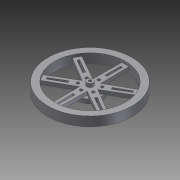
# Autodesk Inventor part: Wheel90mm
Saved by Autodesk Inventor 2011 SP2 (Build 150309200, 309)
## iProperties
Created: 2015-10-13
Part Number: Wheel90mm
Document SubType Name: Modeling
Designer: Ernest
Density: 1 g/cm^3
Author: Ernest
Autodesk Inventor part; units mm, degrees
ref_plane "YZ Plane" through (0, 0, 0) normal (1, 0, 0) x (0, 1, 0)
ref_plane "XZ Plane" through (0, 0, 0) normal (0, 1, 0) x (-1, 0, 0)
ref_plane "XY Plane" through (0, 0, 0) normal (0, 0, 1) x (1, 0, 0)
sketch "Sketch1" plane through (0, 0, 0) normal (0, 0, 1) x (1, 0, 0)
  circle A0 centre (0, 0) radius 45
  circle A1 centre (0, 0) radius 38
  line L0 (0, 0) -> (0, -38) construction
  line L1 (-1.25, -17) -> (1.25, -17)
  line L2 (1.25, -17) -> (1.05, -34)
  line L3 (1.05, -34) -> (-1.05, -34)
  line L4 (-1.25, -17) -> (-1.05, -34)
  circle A2 centre (0, 0) radius 1.5
  circle A3 centre (0, -9.53) radius 1.6035
  circle A4 centre (8.2532, -4.765) radius 1.6035
  circle A5 centre (8.2532, 4.765) radius 1.6035
  circle A6 centre (0, 9.53) radius 1.6035
  circle A7 centre (-8.2532, 4.765) radius 1.6035
  circle A8 centre (-8.2532, -4.765) radius 1.6035
  line L5 (0, -9.53) -> (8.2532, -4.765) construction
  line L6 (4.1266, -7.1475) -> (3.7658, -37.8129)
  line L7 (0, -9.53) -> (-8.2532, -4.765) construction
  line L8 (-4.1266, -7.1475) -> (-3.7658, -37.8129)
  line L9 (14.0974, -9.5825) -> (15.3474, -7.4175)
  line L10 (15.3474, -7.4175) -> (29.9699, -16.0907)
  line L11 (29.9699, -16.0907) -> (28.9199, -17.9093)
  line L12 (14.0974, -9.5825) -> (28.9199, -17.9093)
  line L13 (8.2532, 0) -> (34.6299, -15.6452)
  line L14 (4.1266, -7.1475) -> (30.864, -22.1678)
  line L15 (15.3474, 7.4175) -> (14.0974, 9.5825)
  line L16 (14.0974, 9.5825) -> (28.9199, 17.9093)
  line L17 (28.9199, 17.9093) -> (29.9699, 16.0907)
  line L18 (15.3474, 7.4175) -> (29.9699, 16.0907)
  line L19 (4.1266, 7.1475) -> (30.864, 22.1678)
  line L20 (8.2532, 0) -> (34.6299, 15.6452)
  line L21 (1.25, 17) -> (-1.25, 17)
  line L22 (-1.25, 17) -> (-1.05, 34)
  line L23 (-1.05, 34) -> (1.05, 34)
  line L24 (1.25, 17) -> (1.05, 34)
  line L25 (-4.1266, 7.1475) -> (-3.7658, 37.8129)
  line L26 (4.1266, 7.1475) -> (3.7658, 37.8129)
  line L27 (-14.0974, 9.5825) -> (-15.3474, 7.4175)
  line L28 (-15.3474, 7.4175) -> (-29.9699, 16.0907)
  line L29 (-29.9699, 16.0907) -> (-28.9199, 17.9093)
  line L30 (-14.0974, 9.5825) -> (-28.9199, 17.9093)
  line L31 (-8.2532, 0) -> (-34.6299, 15.6452)
  line L32 (-4.1266, 7.1475) -> (-30.864, 22.1678)
  line L33 (-15.3474, -7.4175) -> (-14.0974, -9.5825)
  line L34 (-14.0974, -9.5825) -> (-28.9199, -17.9093)
  line L35 (-28.9199, -17.9093) -> (-29.9699, -16.0907)
  line L36 (-15.3474, -7.4175) -> (-29.9699, -16.0907)
  line L37 (-4.1266, -7.1475) -> (-30.864, -22.1678)
  line L38 (-8.2532, 0) -> (-34.6299, -15.6452)
  line L39 (3.7658, -37.8129) -> (4.1266, -7.1475)
  line L40 (30.864, -22.1678) -> (4.1266, -7.1475)
  arc A9 (-30.864, -22.1678) -> (-3.7658, -37.8129) centre (0, 0) ccw
  arc A10 (3.7658, -37.8129) -> (30.864, -22.1678) centre (0, 0) ccw
  line L41 (-30.864, -22.1678) -> (-4.1266, -7.1475)
  line L42 (-4.1266, -7.1475) -> (-3.7658, -37.8129)
  line L43 (-34.6299, -15.6452) -> (-8.2532, 0)
  line L44 (-34.6299, 15.6452) -> (-8.2532, 0)
  line L45 (-4.1266, 7.1475) -> (-30.864, 22.1678)
  line L46 (-4.1266, 7.1475) -> (-3.7658, 37.8129)
  line L47 (4.1266, 7.1475) -> (3.7658, 37.8129)
  line L48 (4.1266, 7.1475) -> (30.864, 22.1678)
  line L49 (34.6299, 15.6452) -> (8.2532, 0)
  line L50 (8.2532, 0) -> (34.6299, -15.6452)
  arc A11 (-34.6299, 15.6452) -> (-34.6299, -15.6452) centre (0, 0) ccw
  arc A12 (-3.7658, 37.8129) -> (-30.864, 22.1678) centre (0, 0) ccw
  arc A13 (30.864, 22.1678) -> (3.7658, 37.8129) centre (0, 0) ccw
  arc A14 (34.6299, -15.6452) -> (34.6299, 15.6452) centre (0, 0) ccw
  arc A15 (-3.7658, 37.8129) -> (-30.864, 22.1678) centre (0, 0) ccw
  arc A16 (-3.7658, 37.8129) -> (-30.864, 22.1678) centre (0, 0) ccw
  line L51 (-30.864, 22.1678) -> (-4.1266, 7.1475)
  line L52 (-4.1266, 7.1475) -> (-3.7658, 37.8129)
  point P0 (32.909, -19)
  point P1 (8.2532, -4.765)
  point P2 (32.909, 19)
  point P3 (8.2532, 4.765)
  point P4 (0, 38)
  point P5 (0, 9.53)
  point P6 (-32.909, 19)
  point P7 (-8.2532, 4.765)
  point P8 (-32.909, -19)
  point P9 (-8.2532, -4.765)
  dimension "d0" = 90
  dimension "d1" = 76
  dimension "d2" = 2.1
  dimension "d3" = 2.5
  dimension "d4" = 1.25
  dimension "d5" = 1.05
  dimension "d6" = 3
  dimension "d7" = 17
  dimension "d8" = 4
  dimension "d9" = 9.53
  dimension "d12" = 360
  dimension "d16" = 360
  dimension "d20" = 3.207
  constraints: 106 end point, 20 point on circle, 17 centre point, 13 collinear, 8 concentric, 3 coincident, 2 midpoint, 2 parallel, 2 perpendicular, 1 point on line, 1 vertical, 110 other
  measures "d0" diameter of A0
  measures "d1" diameter of A1
  measures "d2" distance of L2.end L3.end
  measures "d3" distance of L1.end L1.start
  measures "d4" distance from line of L0 L1.end
  measures "d5" distance from line of L3.end L0
  measures "d6" diameter of A2
  measures "d7" distance between parallel lines of L3 L1
  measures "d8" distance from line of L0.end L3
  measures "d9" distance of point (0, 0) L5.start
  measures "d20" diameter of A5
extrude "Extrusion1" add sketch "Sketch1" along normal mid plane 10 contours A0
extrude "Extrusion2" add sketch "Sketch1" along normal mid plane 4 contours L20 L13 A1 L14 L6 L8 L37 L38 L31 L32 L25 L26 L19
sketch "Sketch2" plane through (0, 0, 2) normal (0, 0, 1) x (1, 0, 0)
  circle A0 centre (0, 0) radius 1.5 projected
  circle A1 centre (0, 0) radius 3.5
  dimension "d23" = 7
  constraints: 1 centre point, 1 coincident
  measures "d23" diameter of A1
extrude "Extrusion3" add sketch "Sketch2" along normal blind 3.9
sketch "Sketch3" plane through (0, 0, -2) normal (0, 0, -1) x (-1, 0, 0)
  circle A0 centre (8.2532, -4.765) radius 1.6035 projected
  circle A1 centre (8.2532, 4.765) radius 1.6035 projected
  circle A2 centre (0, 9.53) radius 1.6035 projected
  circle A3 centre (-8.2532, 4.765) radius 1.6035 projected
  circle A4 centre (-8.2532, -4.765) radius 1.6035 projected
  circle A5 centre (0, -9.53) radius 1.6035 projected
  circle A6 centre (0, 0) radius 1.5 projected
  circle A7 centre (0, 0) radius 12.7
  circle A8 centre (0, 0) radius 3.5 projected
  circle A9 centre (0, 0) radius 3
  circle A10 centre (0, 0) radius 5.5
  dimension "d26" = 6
  dimension "d27" = 11
  dimension "d28" = 25.4
  constraints: 3 centre point, 3 coincident
  measures "d26" diameter of A9
  measures "d27" diameter of A10
  measures "d28" diameter of A7
extrude "Extrusion4" add sketch "Sketch3" along normal blind 4.6 contours A7
extrude "Extrusion5" add sketch "Sketch3" along normal blind 9.2 contours A8 | A10
body "Solid1"
